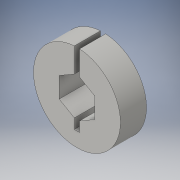
# Autodesk Inventor part: Collar
Saved by Autodesk Inventor 2016 SP2 (Build 200236200, 236)
## iProperties
Created: 2018-01-13
Part Number: Collar
Material: Generic
Document SubType Name: Modeling
Designer: CAD
Density: 1 g/cm^3
Appearance: Default
Author: CAD
Autodesk Inventor part; units mm, degrees
ref_plane "YZ Plane" through (0, 0, 0) normal (1, 0, 0) x (0, 1, 0)
ref_plane "XZ Plane" through (0, 0, 0) normal (0, 1, 0) x (-1, 0, 0)
ref_plane "XY Plane" through (0, 0, 0) normal (0, 0, 1) x (1, 0, 0)
sketch "Sketch1" plane through (0, 0, 0) normal (0, 0, 1) x (1, 0, 0)
  circle A0 centre (0, 0) radius 15.875
  dimension "d0" = 31.75
  constraints: 1 centre point, 1 coincident
  measures "d0" diameter of A0
extrude "Extrusion1" add sketch "Sketch1" along normal blind 9.525
sketch "Sketch2" plane through (0, 0, 9.525) normal (0, 0, 1) x (1, 0, 0)
  line L0 (-6.477, -3.7395) -> (-6.477, 3.7395)
  line L1 (-6.477, 3.7395) -> (0, 7.479)
  line L2 (0, 7.479) -> (6.477, 3.7395)
  line L3 (6.477, 3.7395) -> (6.477, -3.7395)
  line L4 (6.477, -3.7395) -> (0, -7.479)
  line L5 (0, -7.479) -> (-6.477, -3.7395)
  circle A0 centre (0, 0) radius 15.875 projected
  line L6 (-0.9525, 15.8464) -> (-0.9525, -10.5696)
  line L7 (-0.9525, -10.5696) -> (0.9525, -10.5696)
  line L8 (0.9525, -10.5696) -> (0.9525, 15.8464)
  arc A1 (0.9525, 15.8464) -> (-0.9525, 15.8464) centre (0, 0) ccw
  point P0 (-6.477, 0)
  dimension "d3" = 12.954
  dimension "d4" = 1.905
  dimension "d5" = 0.9525
  dimension "d6" = 26.416
  constraints: 18 end point, 4 point on circle, 2 perpendicular, 2 vertical, 1 centre point, 1 coincident, 1 concentric, 1 midpoint, 13 other
  measures "d3" distance between parallel lines of L3 L0
  measures "d4" distance between parallel lines of L8 L6
  measures "d5" distance from line of L4.end L8
  measures "d6" distance of L7.end L8.end
extrude "Extrusion2" cut sketch "Sketch2" against normal blind 9.525 contours L0 L1 L6 L5 | L6 L1 L2 L8 L4 L5 | L5 L4 L8 L7 L6 | L6 A0 L8 L2 L1 | L8 L2 L3 L4
equation "\"d5\" = 0.5 * d4"
body "Solid1"
